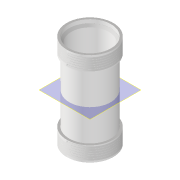
# Autodesk Inventor part: 00_Compression_Coupling_3inch_KingBrothers_CPC-3000
Saved by Autodesk Inventor 2022 (Build 260153000, 153)
## iProperties
Created: 2022-04-19
Part Number: 00_Compression_Coupling_3inch_KingBrothers_CPC-3000
Material: Generic
Document SubType Name: Modeling
Designer: Prakash Lab
Density: 1 g/cm^3
Appearance: Default
Author: Prakash Lab
Autodesk Inventor part; units mm, degrees
ref_plane "YZ Plane" through (0, 0, 0) normal (1, 0, 0) x (0, 1, 0)
ref_plane "XZ Plane" through (0, 0, 0) normal (0, 1, 0) x (-1, 0, 0)
ref_plane "XY Plane" through (0, 0, 0) normal (0, 0, 1) x (1, 0, 0)
sketch "Sketch1" plane through (0, 0, 0) normal (0, 1, 0) x (-1, 0, 0)
  circle A0 centre (0, 0) radius 50.8
  circle A1 centre (0, 0) radius 45.75
  dimension "d0" = 101.6
  dimension "d1" = 91.5
  constraints: 2 centre point, 2 coincident
  measures "d0" diameter of A0
  measures "d1" diameter of A1
extrude "Extrusion1" add sketch "Sketch1" along normal blind 153
sketch "Sketch2" plane through (0, 153, 0) normal (0, 1, 0) x (1, 0, 0)
  circle A0 centre (0, 0) radius 50.8 projected
  circle A1 centre (0, 0) radius 45.75 projected
  circle A2 centre (0, 0) radius 56.28
  circle A3 centre (0, 0) radius 45.75 projected
  dimension "d4" = 112.56
  constraints: 1 centre point, 1 coincident
  measures "d4" diameter of A2
extrude "Extrusion2" add sketch "Sketch2" along normal blind 36.42 contours A0 | A2
sketch "Sketch3" plane through (0, 189.42, 0) normal (0, 1, 0) x (1, 0, 0)
  circle A0 centre (0, 0) radius 50.925
  dimension "d7" = 101.85
  constraints: 1 centre point, 1 coincident
  measures "d7" diameter of A0
extrude "Extrusion3" cut sketch "Sketch3" against normal blind 8.64
chamfer "Chamfer1" distance 5 angle 45 1 edges at (-45.75, 180.78, 0)
sketch "Sketch4" plane through (0, 0, 0) normal (1, 0, 0) x (0, 1, 0)
  line L0 (189.42, -56.28) -> (189.42, 56.28) projected
  line L1 (189.42, 56.28) -> (186.9388, 53.8903)
  line L2 (186.9388, 53.8903) -> (184.6373, 56.28)
  line L3 (153, 56.28) -> (189.42, 56.28) projected
  line L4 (189.42, 56.28) -> (184.6373, 56.28)
  point P0 (0, 0)
  constraints: 6 end point, 1 horizontal, 1 perpendicular, 1 point on line
coil "Coil1" sketch "Sketch4" operation cut axis through (0, -10, 0) along (0, -1, 0) pitch 5 turns 6 hand right
ref_plane "Work Plane1" through (0, 76.5, 0) normal (0, -1, 0) x (1, 0, 0)
mirror "Mirror1" about plane through (0, 76.5, 0) normal (0, -1, 0) of "Extrusion2", "Extrusion3", "Chamfer1", "Coil1"
body "Solid1"
